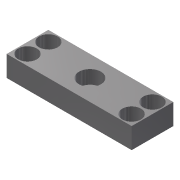
# Autodesk Inventor part: GARFO
Saved by Autodesk Inventor 2015 (Build 190159000, 159)
## iProperties
Created: 2016-08-09
Part Number: GARFO
Material: Aluminium AW-7020
Document SubType Name: Modeling
Designer: EriveltonDell
Density: 2.78 g/cm^3
Appearance: Stainless - Brushed
Mass: 1234.07 g
Surface Area: 731.335 cm^2
Volume: 443.911 cm^3
Author: EriveltonDell
Autodesk Inventor part; units mm, degrees
ref_plane "YZ Plane" through (0, 0, 0) normal (1, 0, 0) x (0, 1, 0)
ref_plane "XZ Plane" through (0, 0, 0) normal (0, 1, 0) x (-1, 0, 0)
ref_plane "XY Plane" through (0, 0, 0) normal (0, 0, 1) x (1, 0, 0)
sketch "Sketch4" plane through (0, 0, 0) normal (0, 0, 1) x (1, 0, 0)
  line L0 (0, 0) -> (-60, 0)
  line L1 (-60, 0) -> (-60, 20)
  line L2 (-60, 20) -> (0, 20)
  line L3 (0, 20) -> (0, 0)
  dimension "d37" = 60
  dimension "d38" = 20
  constraints: 8 end point, 2 parallel, 1 horizontal, 1 perpendicular
  measures "d37" distance of L1.end L2.end
  measures "d38" distance of L0.end L1.end
extrude "Extrusion2" add sketch "Sketch4" along normal blind 10
hole "Hole2" at (-30, 10, 10) direction (0, 0, -1) diameter 6.5 depth 10 tip angle 118 counterbore diameter 10.5 counterbore depth 6.5
hole "Hole3" at (-55, 15, 10) direction (0, 0, -1) diameter 5.5 depth 10 tip angle 118 counterbore diameter 9 counterbore depth 8
hole "Hole4" at (-5, 15, 10) direction (0, 0, -1) diameter 5.5 depth 10 tip angle 118 counterbore diameter 9 counterbore depth 8
hole "Hole5" at (-5, 5, 10) direction (0, 0, -1) diameter 5.5 depth 10 tip angle 118 counterbore diameter 9 counterbore depth 8
hole "Hole6" at (-55, 5, 10) direction (0, 0, -1) diameter 5.5 depth 10 tip angle 118 counterbore diameter 9 counterbore depth 8
body "Solid2"
